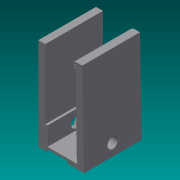
# Autodesk Inventor part: MotorClip
Saved by Autodesk Inventor 2013 (Build 170138000, 138)
## iProperties
Created: 2013-08-16
Part Number: MotorClip
Material: Generic
Document SubType Name: Modeling
Designer: Sawaiz
Density: 1 g/cm^3
Author: Sawaiz
Autodesk Inventor part; units mm, degrees
ref_plane "YZ Plane" through (0, 0, 0) normal (1, 0, 0) x (0, 1, 0)
ref_plane "XZ Plane" through (0, 0, 0) normal (0, 1, 0) x (-1, 0, 0)
ref_plane "XY Plane" through (0, 0, 0) normal (0, 0, 1) x (1, 0, 0)
sketch "Sketch1" plane through (0, 0, 0) normal (1, 0, 0) x (0, 1, 0)
  line L0 (0, 0) -> (40, -0.6982)
  line L1 (40, -0.6982) -> (39.9486, -3.6454)
  line L2 (39.9486, -3.6454) -> (36.9486, -3.6454)
  line L3 (36.9486, -3.6454) -> (2, -3.0354)
  line L4 (2, -3.0354) -> (2, -16.7514)
  line L5 (2, -16.7514) -> (40, -16.7514)
  line L6 (40, -16.7514) -> (40, -19.7514)
  line L7 (40, -19.7514) -> (0, -19.7514)
  line L8 (0, -19.7514) -> (0, 0)
  line L9 (10, -16.7514) -> (10, -15.7514)
  line L10 (10, -15.7514) -> (2, -15.7514)
  line L11 (39.9486, -3.6454) -> (39.4486, -4.5114)
  line L12 (39.9486, -3.6454) -> (40.9486, -3.6454) construction
  line L13 (39.4486, -4.5114) -> (38.9486, -3.6454)
  line L14 (36.9486, -3.6454) -> (37.4486, -4.5114)
  line L15 (37.4486, -4.5114) -> (37.9486, -3.6454)
  line L16 (37.9486, -3.6454) -> (38.4486, -4.5114)
  line L17 (38.4486, -4.5114) -> (38.9486, -3.6454)
  line L18 (0, -5.2681) -> (1, -5.2681)
  line L19 (1, -5.2681) -> (1, -14.2681)
  line L20 (1, -14.2681) -> (0, -14.2681)
  dimension "d5" = 40
  dimension "d6" = 13.716
  dimension "d7" = 3
  dimension "d8" = 3
  dimension "d9" = 40
  dimension "d10" = 3
  dimension "d11" = 2
  dimension "d12" = 89
  dimension "d13" = 1
  dimension "d14" = 30
  dimension "d15" = 1
  dimension "d16" = 120
  dimension "d17" = 120
  dimension "d18" = 60
  dimension "d19" = 60
  dimension "d20" = 1
  dimension "d33" = 1
  dimension "d34" = 9
  constraints: 42 end point, 9 perpendicular, 6 parallel, 6 point on line, 2 horizontal, 1 equal length
  measures "d5" distance of L6.end L7.end
  measures "d6" distance of L3.end L4.end
  measures "d7" distance between parallel lines of L7 L5
  measures "d8" distance between parallel lines of L0 L3
  measures "d9" horizontal distance of L0.start L0.end
  measures "d10" distance of L1.end L2.end
  measures "d11" distance between parallel lines of L8 L4
  measures "d12" angle of L8 L0
  measures "d13" distance of L9.start L9.end
  measures "d14" distance between parallel lines of L6 L9
  measures "d15" distance of L1.end L11.end
  measures "d16" angle of L11 L12
  measures "d17" angle of L2 L13
  measures "d18" angle of L2 L14
  measures "d19" angle of L15 L2
  measures "d20" distance of L14.end L15.end
  measures "d33" distance of L18.start L18.end
  measures "d34" distance of L18.end L19.end
extrude "Extrusion1" add sketch "Sketch1" along normal blind 25
sketch "Sketch2" plane through (0, 0, -19.7514) normal (0, 0, -1) x (-1, 0, 0)
  line L0 (0, 10) -> (-25, 10) projected
  line L1 (-25, 10) -> (0, 0)
  line L2 (-7.459, 5) -> (-9.9795, 0.6344)
  line L3 (-9.9795, 0.6344) -> (-15.0205, 0.6344)
  line L4 (-15.0205, 0.6344) -> (-17.541, 5)
  line L5 (-17.541, 5) -> (-15.0205, 9.3656)
  line L6 (-15.0205, 9.3656) -> (-9.9795, 9.3656)
  line L7 (-9.9795, 9.3656) -> (-7.459, 5)
  point P0 (-12.5, 5)
  dimension "d23" = 8.7312
  constraints: 14 end point, 1 midpoint, 13 other
  measures "d23" distance between parallel lines of L2 L5
extrude "Extrusion2" cut sketch "Sketch2" against normal blind 3.175
sketch "Sketch3" plane through (0, 0, -16.5764) normal (0, 0, -1) x (-1, 0, 0)
  point P0 (0, 0)
  point P1 (-12.5, 5)
hole "Hole1" at (12.5, 5, -16.5764) direction (0, 0, 1) diameter 4.4958 end through all
sketch "Sketch4" plane through (0, 0, 0) normal (-1, 0, 0) x (0, 0, 1)
  line L0 (-19.7514, 0) -> (-19.7514, 40) projected
  line L1 (0, 0) -> (-19.7514, 0) projected
  line L2 (-7.2514, 0) -> (-16.2514, 0)
  line L3 (-16.2514, 0) -> (-16.2514, 1)
  line L4 (-16.2514, 1) -> (-7.2514, 1)
  line L5 (-7.2514, 1) -> (-7.2514, 0)
  dimension "d35" = 9
  dimension "d36" = 1
  dimension "d38" = 3.5
  constraints: 8 end point, 2 parallel, 1 horizontal, 1 perpendicular, 1 point on line
  measures "d35" distance of L3.end L4.end
  measures "d36" distance of L2.end L3.end
  measures "d38" distance between parallel lines of L0 L3
extrude "Extrusion3" cut sketch "Sketch4" against normal through all
equation "\"d6\" = StretcherDepth"
equation "\"d8\" = d7"
equation "\"d9\" = d5"
equation "\"StretcherDepth\" = 13.716"
body "Solid1"
